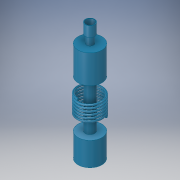
# Autodesk Inventor part: minifridge
Saved by Autodesk Inventor 2018 (Build 220112000, 112)
## iProperties
Created: 2019-03-15
Part Number: minifridge
Material: Brass, Soft Yellow
Document SubType Name: Modeling
Designer: Admin
Density: 8.47 g/cm^3
Appearance: Sky Blue Dark
Author: Admin
Autodesk Inventor part; units mm, degrees
ref_plane "YZ Plane" through (0, 0, 0) normal (1, 0, 0) x (0, 1, 0)
ref_plane "XZ Plane" through (0, 0, 0) normal (0, 1, 0) x (-1, 0, 0)
ref_plane "XY Plane" through (0, 0, 0) normal (0, 0, 1) x (1, 0, 0)
sketch "Sketch3" plane through (0, 0, 0) normal (0, 1, 0) x (-1, 0, 0)
  circle A0 centre (0, 0) radius 5.588
  circle A1 centre (0, 0) radius 6.35
  dimension "d6" = 11.176
  dimension "d7" = 12.7
  constraints: 2 centre point, 2 coincident
  measures "d6" diameter of A0
  measures "d7" diameter of A1
extrude "Extrusion3" add sketch "Sketch3" along normal blind 11.176
sketch "Sketch4" plane through (0, 0, 0) normal (0, -1, 0) x (1, 0, 0)
  circle A0 centre (0, 0) radius 3.81
  circle A1 centre (0, 0) radius 6.35
  circle A2 centre (0, 0) radius 6.35 projected
  dimension "d10" = 7.62
  constraints: 2 centre point, 2 coincident, 1 concentric
  measures "d10" diameter of A0
extrude "Extrusion4" add sketch "Sketch4" along normal blind 2.54
sketch "Sketch5" plane through (0, -2.54, 0) normal (0, -1, 0) x (1, 0, 0)
  circle A0 centre (0, 0) radius 3.81
  circle A1 centre (0, 0) radius 4.572
  circle A2 centre (0, 0) radius 3.81 projected
  dimension "d13" = 0.762
  constraints: 2 centre point, 2 coincident, 1 concentric
  measures "d13" radial gap between concentric circles of A0 A1
extrude "Extrusion5" add sketch "Sketch5" along normal blind 11.176
sketch "Sketch6" plane through (0, -13.716, 0) normal (0, -1, 0) x (1, 0, 0)
  circle A0 centre (0, 0) radius 15.875
  dimension "d16" = 31.75
  constraints: 1 centre point, 1 coincident
  measures "d16" diameter of A0
extrude "Extrusion6" add sketch "Sketch6" along normal blind 38.1
sketch "Sketch7" plane through (0, -51.816, 0) normal (0, -1, 0) x (1, 0, 0)
  circle A0 centre (0, 0) radius 6.35
  dimension "d19" = 12.7
  constraints: 1 centre point, 1 coincident
  measures "d19" diameter of A0
extrude "Extrusion7" add sketch "Sketch7" along normal blind 63.5
sketch "Sketch8" plane through (0, 0, 0) normal (1, 0, 0) x (0, 1, 0)
  line L0 (-115.316, 6.35) -> (-115.316, -6.35) projected
  circle A0 centre (-70.866, 15.875) radius 1.27
  line L1 (-51.816, 15.875) -> (-51.816, -15.875) projected
  line L2 (-51.816, 0) -> (-70.866, 0)
  line L3 (-70.866, 0) -> (-70.866, 15.875)
  point P0 (0, 0)
  dimension "d23" = 2.54
  dimension "d32" = 15.875
  dimension "d33" = 19.05
  constraints: 4 end point, 1 centre point, 1 coincident, 1 horizontal, 1 midpoint, 1 perpendicular
  measures "d23" diameter of A0
  measures "d32" distance of L2.end L3.end
  measures "d33" distance of L2.start L2.end
coil "Coil1" sketch "Sketch8" operation add axis through (0, -10, 0) along (0, -1, 0) pitch 3.81 turns 6.666667 hand right
sketch "Sketch9" plane through (0, -115.316, 0) normal (0, -1, 0) x (1, 0, 0)
  circle A0 centre (0, 0) radius 3.81 projected
  circle A1 centre (0, 0) radius 15.875
  dimension "d34" = 31.75
  constraints: 1 centre point, 1 coincident
  measures "d34" diameter of A1
extrude "Extrusion8" add sketch "Sketch9" along normal blind 31.75
body "Solid2"
